ikea-stolmen-hook-two-pieces (Autodesk Fusion 360 design; units mm, degrees)
Autodesk Fusion 360 part; units mm, degrees
sketch "Sketch1" plane through (0, 0, 0) normal (0, 1, 0) x (1, 0, 0) in component "Component"
  circle A0 centre (0, 0) radius 23.5
  circle A1 centre (0, 0) radius 27.5
  line L0 (-5, 35.5) -> (-9, 35.5)
  line L1 (-9, 35.5) -> (-9, 23.5)
  line L2 (-9, 23.5) -> (-5, 23.5)
  line L3 (-5, 23.5) -> (-5, 35.5)
  line L4 (0, 5) -> (0, -5)
  line L5 (-5, 0) -> (5, 0)
  line L6 (9, 35.5) -> (9, 23.5)
  line L7 (5, 23.5) -> (5, 35.5)
  line L8 (9, 23.5) -> (5, 23.5)
  line L9 (5, 35.5) -> (9, 35.5)
  line L10 (-5, 23.5) -> (-5, -23.5)
  line L11 (5, -23.5) -> (5, 23.5)
  circle A2 centre (0, 0) radius 25
  circle A3 centre (0, 0) radius 26
  line L12 (-30, 5) -> (-20, 5)
  line L13 (30, 5) -> (20, 5)
  line L14 (-30, -5) -> (-20, -5)
  line L15 (30, -5) -> (20, -5)
  dimension "d2" = 47
  dimension "d4" = 55
  dimension "d7" = 4
  dimension "d54" = 12
  measures "d2" diameter of A0
  measures "d4" diameter of A1
  measures "d7" distance of L0.start L0.end
  measures "d54" distance of L0.end L1.end
extrude "Extrude1" add sketch "Sketch1" along normal blind 8 contours A0 L8 L11 A2 L13 | A0 A2 L14 L15 | A2 A3 L13 L15 | L6 L8 A2 A3 L13 | A2 A3 L14 L15 | A0 L2 L10 A2 L12 | L7 L8 A2 | L6 L7 L8 A2 A3 | A1 L6 A3 L13 | A2 A3 L12 L14 | A1 A3 L14 L15 | L2 L3 A2 | A1 L6 L7 A3 | L1 L2 A2 A3 L12 | L1 L2 L3 A2 A3 | A1 L6 L7 L9 | A1 L1 A3 L12 | A1 L1 L3 A3 | A1 L0 L1 L3 makes body 1 in component "Component"
fillet "Fillet6" radius 4 2 edges at (7, 8, -35.5) (7, 0, -35.5) on bodies 1 in component "Component"
fillet "Fillet6" radius 4 2 edges at (-7, 8, -35.5) (-7, 0, -35.5) on bodies 1 in component "Component"
sketch "Sketch6" plane through (-9, 0, 0) normal (-1, 0, 0) x (0, 0, 1)
  arc A0 (-31.5, 8) -> (-31.5, 0) centre (-31.5, 4) ccw
  line L0 (-31.5, 0) -> (-25.9856, 0)
  line L1 (-25.9856, 0) -> (-25.9856, 8)
  line L2 (-25.9856, 8) -> (-31.5, 8)
  circle A1 centre (-31.5, 4) radius 1.6
  line L3 (-31.5, 7.1) -> (-34.1847, 5.55)
  line L4 (-34.1847, 5.55) -> (-34.1847, 2.45)
  line L5 (-34.1847, 2.45) -> (-31.5, 0.9)
  line L6 (-31.5, 0.9) -> (-28.8153, 2.45)
  line L7 (-28.8153, 2.45) -> (-28.8153, 5.55)
  line L8 (-28.8153, 5.55) -> (-31.5, 7.1)
  point P0 (-31.5, 4)
  dimension "d73" = 3.2
  measures "d73" diameter of A1
extrude "Extrude8" cut sketch "Sketch6" against normal up to surface (18 mm away) contours A1 bodies 1 in component "Component"
extrude "Extrude9" cut sketch "Sketch6" against normal blind 1 contours L3 L4 L5 L6 L7 L8 bodies 1 in component "Component"
fillet "Fillet8" radius 4 16 edges at (24.4949, 4, 5) (22.9619, 4, 5) (22.9619, 4, -5) (24.4949, 4, -5) (25.5147, 4, -5) (27.0416, 4, -5) (27.0416, 4, 5) (-27.0416, 4, -5) (-27.0416, 4, 5) (-25.5147, 4, 5) (-22.9619, 4, 5) (-22.9619, 4, -5) (-24.4949, 4, -5) (-25.5147, 4, -5) (-24.4949, 4, 5) (25.5147, 4, 5) on bodies 1 in component "Component"
sketch "Sketch5" plane through (0, 0, 0) normal (0, 1, 0) x (1, 0, 0)
  circle A0 centre (-14.9966, 15) radius 4
  line L0 (-18.9966, 15) -> (-18.9966, 0)
  line L1 (-10.9966, 15) -> (-10.9966, 0)
  arc A1 (-35, 0) -> (-18.9966, 0) centre (-26.9983, 0) ccw
  arc A2 (-43, 0) -> (-10.9966, 0) centre (-26.9983, 0) ccw
  circle A3 centre (-39, 0) radius 4
  circle A4 centre (-14.9966, 15) radius 1.6
  line L2 (-14.9966, 2) -> (-6.4966, 2)
  line L3 (-6.4966, 2) -> (-6.4966, -2)
  line L4 (-6.4966, -2) -> (-14.9966, -2)
  line L5 (-14.9966, -2) -> (-14.9966, 2)
  line L6 (-18.9966, 0) -> (-10.9966, 0)
  dimension "d64" = 8
  dimension "d65" = 8
  dimension "d66" = 8
  dimension "d67" = 3.2
  dimension "d68" = 8.5
  measures "d64" diameter of A0
  measures "d65" distance of L0.end L1.end
  measures "d66" distance of A1.start A2.start
  measures "d67" diameter of A4
  measures "d68" distance of L3.end L4.end
extrude "Extrude2" add sketch "Sketch5" along normal blind 10 separate body makes body 2
fillet "Fillet4" radius 3 2 edges at (-11.1221, 5, 2) (-10.9966, 5, -2) on bodies 2
component "Component" placed x (1, 0, 0) y (0, 1, 0) z (0, 0, 1) at (0, 0, 0)
equation "ikeaStolmanPoleDiameter = 47 mm"
equation "d2 = ikeaStolmanPoleDiameter"
equation "thickness = 4 mm"
equation "d4 = ikeaStolmanPoleDiameter + thickness + thickness"
equation "d7 = thickness"
equation "d11 = height"
equation "flexThickness = 0.75 mm"
equation "height = 8 mm"
equation "d55 = thickness"
equation "d64 = height"
equation "d66 = height"
equation "d72 = thickness"
